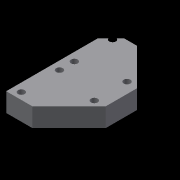
# Autodesk Inventor part: AX_XY
Saved by Autodesk Inventor 2016 (Build 200138000, 138)
## iProperties
Created: 2017-08-22
Part Number: AX_XY
Material: PC/ABS Plastic
Document SubType Name: Modeling
Designer: ludwi
Density: 0.357273 g/cm^3
Appearance: Smooth - White
Author: ludwi
Autodesk Inventor part; units mm, degrees
ref_plane "YZ Plane" through (0, 0, 0) normal (1, 0, 0) x (0, 1, 0)
ref_plane "XZ Plane" through (0, 0, 0) normal (0, 1, 0) x (-1, 0, 0)
ref_plane "XY Plane" through (0, 0, 0) normal (0, 0, 1) x (1, 0, 0)
sketch "Sketch1" plane through (0, 0, 0) normal (0, 0, 1) x (1, 0, 0)
  line L0 (-58, -50) -> (-58, 50) construction
  line L1 (-58, -50) -> (58, -50) construction
  line L2 (58, 50) -> (58, -50) construction
  line L3 (58, 50) -> (-58, 50) construction
  line L4 (-48.8, -35) -> (-48.8, -43.5) construction
  arc A0 (-55.2, -43.5) -> (-48.8, -43.5) centre (-52, -43.5) ccw construction
  line L5 (-55.2, -43.5) -> (-55.2, -35) construction
  arc A1 (-48.8, -35) -> (-55.2, -35) centre (-52, -35) ccw construction
  line L6 (55.2, -35) -> (55.2, -43.5) construction
  arc A2 (48.8, -43.5) -> (55.2, -43.5) centre (52, -43.5) ccw construction
  line L7 (48.8, -43.5) -> (48.8, -35) construction
  arc A3 (55.2, -35) -> (48.8, -35) centre (52, -35) ccw construction
  circle A4 centre (10.25, -35) radius 3.2 construction
  circle A5 centre (-10.25, -35) radius 3.2 construction
  circle A6 centre (-10.25, 35) radius 3.2 construction
  circle A7 centre (10.25, 35) radius 3.2 construction
  line L8 (-55.2, 35) -> (-55.2, 43.5) construction
  arc A8 (-48.8, 43.5) -> (-55.2, 43.5) centre (-52, 43.5) ccw construction
  line L9 (-48.8, 43.5) -> (-48.8, 35) construction
  arc A9 (-55.2, 35) -> (-48.8, 35) centre (-52, 35) ccw construction
  circle A10 centre (-52, 7.125) radius 3.2 construction
  line L10 (-7.05, -7.125) -> (-7.05, -15.625) construction
  arc A11 (-13.45, -15.625) -> (-7.05, -15.625) centre (-10.25, -15.625) ccw construction
  line L11 (-13.45, -15.625) -> (-13.45, -7.125) construction
  arc A12 (-7.05, -7.125) -> (-13.45, -7.125) centre (-10.25, -7.125) ccw construction
  circle A13 centre (52, -7.125) radius 3.2 construction
  circle A14 centre (-52, -7.125) radius 3.2 construction
  line L12 (13.45, -7.125) -> (13.45, -15.625) construction
  arc A15 (7.05, -15.625) -> (13.45, -15.625) centre (10.25, -15.625) ccw construction
  line L13 (7.05, -15.625) -> (7.05, -7.125) construction
  arc A16 (13.45, -7.125) -> (7.05, -7.125) centre (10.25, -7.125) ccw construction
  circle A17 centre (52, 7.125) radius 3.2 construction
  line L14 (13.45, 15.625) -> (13.45, 7.125) construction
  arc A18 (7.05, 7.125) -> (13.45, 7.125) centre (10.25, 7.125) ccw construction
  line L15 (7.05, 7.125) -> (7.05, 15.625) construction
  arc A19 (13.45, 15.625) -> (7.05, 15.625) centre (10.25, 15.625) ccw construction
  line L16 (55.2, 43.5) -> (55.2, 35) construction
  arc A20 (48.8, 35) -> (55.2, 35) centre (52, 35) ccw construction
  line L17 (48.8, 35) -> (48.8, 43.5) construction
  arc A21 (55.2, 43.5) -> (48.8, 43.5) centre (52, 43.5) ccw construction
  line L18 (-7.05, 15.625) -> (-7.05, 7.125) construction
  arc A22 (-13.45, 7.125) -> (-7.05, 7.125) centre (-10.25, 7.125) ccw construction
  line L19 (-13.45, 7.125) -> (-13.45, 15.625) construction
  arc A23 (-7.05, 15.625) -> (-13.45, 15.625) centre (-10.25, 15.625) ccw construction
  line L20 (60, 50) -> (58, 50) construction
  line L21 (58, 50) -> (58, -50) construction
  line L22 (58, -50) -> (60, -50) construction
  line L23 (60, -50) -> (60, 50) construction
  line L24 (-60, -50) -> (-58, -50) construction
  line L25 (-58, -50) -> (-58, 50) construction
  line L26 (-58, 50) -> (-60, 50) construction
  line L27 (-60, 50) -> (-60, -50) construction
  circle A24 centre (-52, 43.5) radius 3.2
  circle A25 centre (-10.25, 15.625) radius 3.2
  line L28 (0, 50) -> (0, 0) construction
  circle A26 centre (52, 43.5) radius 3.2
  circle A27 centre (10.25, 15.625) radius 3.2
  circle A28 centre (-52, -43.5) radius 3.2
  circle A29 centre (-52, 7.125) radius 3.2
  circle A30 centre (-52, -7.125) radius 3.2
  circle A31 centre (-10.25, -15.625) radius 3.2
  circle A32 centre (-10.25, -35) radius 3.2
  circle A33 centre (-10.25, 35) radius 3.2
  line L29 (-60, 50) -> (-60, -50)
  line L30 (-60, -50) -> (-35, -50)
  line L31 (-35, -50) -> (0, -15)
  line L32 (0, -15) -> (0, 15)
  line L33 (-60, 50) -> (-35, 50)
  line L34 (-35, 50) -> (0, 15)
  dimension "d12" = 45
  dimension "d13" = 35
  constraints: 14 end point, 8 centre point, 8 coincident, 6 concentric, 3 point on line, 3 vertical, 2 horizontal alignment, 2 perpendicular, 2 symmetric about line, 1 midpoint, 6 other
  measures "d12" angle of L3 L34
  measures "d13" horizontal distance of L32.end L33.end
extrude "Extrusion1" add sketch "Sketch1" along normal blind 18 contours L33 L34 L32 L31 L30 L29
sketch "Sketch4" plane through (-60, -50, 0) normal (-1, 0, 0) x (0, 0, 1)
  line L0 (16, 100) -> (16, 0) projected
  line L1 (16, 100) -> (0, 100) projected
  line L2 (0, 88) -> (0, 100) projected
  arc A0 (0, 72) -> (0, 88) centre (0, 80) ccw projected
  line L3 (0, 62.5) -> (0, 72) projected
  arc A1 (0, 37.5) -> (0, 62.5) centre (0, 50) ccw projected
  line L4 (0, 28) -> (0, 37.5) projected
  arc A2 (0, 12) -> (0, 28) centre (0, 20) ccw projected
  line L5 (0, 0) -> (0, 12) projected
  line L6 (16, 0) -> (0, 0) projected
  line L7 (-16, 0) -> (-16, 100) projected
  line L8 (-16, 0) -> (0, 0) projected
  line L9 (0, 12) -> (0, 0) projected
  arc A3 (0, 28) -> (0, 12) centre (0, 20) ccw projected
  line L10 (0, 37.5) -> (0, 28) projected
  arc A4 (0, 62.5) -> (0, 37.5) centre (0, 50) ccw projected
  line L11 (0, 72) -> (0, 62.5) projected
  arc A5 (0, 88) -> (0, 72) centre (0, 80) ccw projected
  line L12 (0, 100) -> (0, 88) projected
  line L13 (-16, 100) -> (0, 100) projected
  circle A6 centre (0, 50) radius 3.3 projected
  point P0 (0, 50)
extrude "Extrusion4" cut sketch "Sketch4" against normal through all contours A0 A5 | A3 A2 | A6
chamfer "Chamfer3" distance 2 angle 45 4 edges at (-60, 0, 18) (-17.5, -32.5, 18) (-17.5, 32.5, 18) (0, 0, 18)
body "Solid1"
